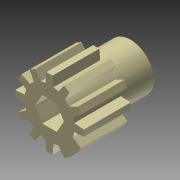
# Autodesk Inventor part: pinion
Saved by Autodesk Inventor 2015 SP1 (Build 190203100, 203)
## iProperties
Created: 2015-01-14
Part Number: pinion
Material: Nylon, molybdenum disulphide
Document SubType Name: Modeling
Designer: Jarod
Density: 1.13 g/cm^3
Appearance: Nylon 6
Author: Jarod
Autodesk Inventor part; units mm, degrees
ref_plane "YZ Plane" through (0, 0, 0) normal (1, 0, 0) x (0, 1, 0)
ref_plane "XZ Plane" through (0, 0, 0) normal (0, 1, 0) x (-1, 0, 0)
ref_plane "XY Plane" through (0, 0, 0) normal (0, 0, 1) x (1, 0, 0)
sketch "Sketch1" plane through (0, 0, 0) normal (0, 0, 1) x (1, 0, 0)
  circle A0 centre (0, 0) radius 11.9062
  dimension "d0" = 23.8125
  constraints: 1 centre point, 1 coincident
  measures "d0" diameter of A0
extrude "Extrusion1" add sketch "Sketch1" along normal blind 41.275
sketch "Sketch2" plane through (0, 0, 41.275) normal (0, 0, 1) x (1, 0, 0)
  circle A0 centre (0, 0) radius 12.7
  dimension "d3" = 25.4
  constraints: 1 centre point, 1 coincident
  measures "d3" diameter of A0
extrude "Extrusion2" add sketch "Sketch2" against normal blind 23.8125
sketch "Sketch3" plane through (0, 0, 41.275) normal (0, 0, 1) x (1, 0, 0)
  line L0 (-3.6662, 6.35) -> (3.6662, 6.35)
  line L1 (3.6662, 6.35) -> (7.3323, 0)
  line L2 (7.3323, 0) -> (3.6662, -6.35)
  line L3 (3.6662, -6.35) -> (-3.6662, -6.35)
  line L4 (-3.6662, -6.35) -> (-7.3323, 0)
  line L5 (-7.3323, 0) -> (-3.6662, 6.35)
  point P0 (0, 0)
  dimension "d6" = 12.7
  dimension "d7" = 12.7
  dimension "d8" = 12.7
  dimension "d9" = 120
  dimension "d10" = 120
  dimension "d11" = 6.35
  dimension "d12" = 6.35
  dimension "d13" = 6.35
  constraints: 12 end point, 3 parallel, 1 horizontal
  measures "d6" distance between parallel lines of L3 L0
  measures "d7" distance between parallel lines of L4 L1
  measures "d8" distance between parallel lines of L2 L5
  measures "d9" angle of L0 L5
  measures "d10" angle of L1 L0
  measures "d11" distance from line of point (0, 0) L0
  measures "d12" distance from line of point (0, 0) L1
  measures "d13" distance from line of point (0, 0) L5
extrude "Extrusion3" cut sketch "Sketch3" against normal blind 50.8
sketch "Sketch4" plane through (0, 0, 41.275) normal (0, 0, 1) x (1, 0, 0)
  line L0 (-7.3323, 0) -> (-3.6662, 6.35) projected
  line L1 (-3.6662, 6.35) -> (3.6662, 6.35) projected
  line L2 (3.6662, 6.35) -> (7.3323, 0) projected
  line L3 (7.3323, 0) -> (3.6662, -6.35) projected
  line L4 (3.6662, -6.35) -> (-3.6662, -6.35) projected
  line L5 (-3.6662, -6.35) -> (-7.3323, 0) projected
  circle A0 centre (0, 0) radius 12.7 projected
  line L6 (0, 12.7) -> (0, 17.4625) construction
  line L7 (0, 12.7) -> (4.7625, 12.7) construction
  line L8 (0, 0) -> (1.9867, 12.5436) construction
  circle A1 centre (0, 0) radius 12.7 construction
  line L9 (0, 0) -> (12.7, 0) construction
  line L10 (0, 0) -> (-1.9867, 12.5436) construction
  line L11 (0, 0) -> (12.7, 0) construction
  line L12 (0, 17.4625) -> (0.7937, 17.4625) construction
  line L13 (0, 17.4625) -> (0.7937, 17.4625) construction
  line L14 (0, 17.4625) -> (-1.5875, 17.4625) construction
  line L15 (0, 17.4625) -> (1.5875, 17.4625) construction
  line L16 (-1.9867, 12.5436) -> (-1.5875, 17.4625)
  line L17 (-1.5875, 17.4625) -> (1.5875, 17.4625)
  line L18 (1.5875, 17.4625) -> (1.9867, 12.5436)
  line L19 (-1.9867, 12.5436) -> (1.9867, 12.5436)
  line L20 (-6.35, 10.9985) -> (-8.7312, 15.123) construction
  line L21 (-6.35, 10.9985) -> (-2.2256, 13.3798) construction
  line L22 (0, 0) -> (-4.5513, 11.8565) construction
  line L23 (0, 0) -> (-7.9924, 9.8698) construction
  line L24 (-8.7312, 15.123) -> (-8.0438, 15.5198) construction
  line L25 (-8.7312, 15.123) -> (-8.0438, 15.5198) construction
  line L26 (-8.7312, 15.123) -> (-10.1061, 14.3292) construction
  line L27 (-8.7312, 15.123) -> (-7.3564, 15.9167) construction
  line L28 (-7.9924, 9.8698) -> (-10.1061, 14.3292)
  line L29 (-10.1061, 14.3292) -> (-7.3564, 15.9167)
  line L30 (-7.3564, 15.9167) -> (-4.5513, 11.8565)
  line L31 (-7.9924, 9.8698) -> (-4.5513, 11.8565)
  line L32 (-10.9985, 6.35) -> (-15.123, 8.7313) construction
  line L33 (-10.9985, 6.35) -> (-8.6173, 10.4744) construction
  line L34 (0, 0) -> (-9.8698, 7.9924) construction
  line L35 (0, 0) -> (-11.8565, 4.5513) construction
  line L36 (-15.123, 8.7313) -> (-14.7261, 9.4187) construction
  line L37 (-15.123, 8.7313) -> (-14.7261, 9.4187) construction
  line L38 (-15.123, 8.7313) -> (-15.9167, 7.3564) construction
  line L39 (-15.123, 8.7313) -> (-14.3292, 10.1061) construction
  line L40 (-11.8565, 4.5513) -> (-15.9167, 7.3564)
  line L41 (-15.9167, 7.3564) -> (-14.3292, 10.1061)
  line L42 (-14.3292, 10.1061) -> (-9.8698, 7.9924)
  line L43 (-11.8565, 4.5513) -> (-9.8698, 7.9924)
  line L44 (-12.7, 0) -> (-17.4625, 0) construction
  line L45 (-12.7, 0) -> (-12.7, 4.7625) construction
  line L46 (0, 0) -> (-12.5436, 1.9867) construction
  line L47 (0, 0) -> (-12.5436, -1.9867) construction
  line L48 (-17.4625, 0) -> (-17.4625, 0.7938) construction
  line L49 (-17.4625, 0) -> (-17.4625, 0.7938) construction
  line L50 (-17.4625, 0) -> (-17.4625, -1.5875) construction
  line L51 (-17.4625, 0) -> (-17.4625, 1.5875) construction
  line L52 (-12.5436, -1.9867) -> (-17.4625, -1.5875)
  line L53 (-17.4625, -1.5875) -> (-17.4625, 1.5875)
  line L54 (-17.4625, 1.5875) -> (-12.5436, 1.9867)
  line L55 (-12.5436, -1.9867) -> (-12.5436, 1.9867)
  line L56 (-10.9985, -6.35) -> (-15.123, -8.7312) construction
  line L57 (-10.9985, -6.35) -> (-13.3798, -2.2256) construction
  line L58 (0, 0) -> (-11.8565, -4.5513) construction
  line L59 (0, 0) -> (-9.8698, -7.9924) construction
  line L60 (-15.123, -8.7312) -> (-15.5198, -8.0438) construction
  line L61 (-15.123, -8.7312) -> (-15.5198, -8.0438) construction
  line L62 (-15.123, -8.7312) -> (-14.3292, -10.1061) construction
  line L63 (-15.123, -8.7312) -> (-15.9167, -7.3564) construction
  line L64 (-9.8698, -7.9924) -> (-14.3292, -10.1061)
  line L65 (-14.3292, -10.1061) -> (-15.9167, -7.3564)
  line L66 (-15.9167, -7.3564) -> (-11.8565, -4.5513)
  line L67 (-9.8698, -7.9924) -> (-11.8565, -4.5513)
  line L68 (-6.35, -10.9985) -> (-8.7313, -15.123) construction
  line L69 (-6.35, -10.9985) -> (-10.4744, -8.6173) construction
  line L70 (0, 0) -> (-7.9924, -9.8698) construction
  line L71 (0, 0) -> (-4.5513, -11.8565) construction
  line L72 (-8.7313, -15.123) -> (-9.4187, -14.7261) construction
  line L73 (-8.7313, -15.123) -> (-9.4187, -14.7261) construction
  line L74 (-8.7313, -15.123) -> (-7.3564, -15.9167) construction
  line L75 (-8.7313, -15.123) -> (-10.1061, -14.3292) construction
  line L76 (-4.5513, -11.8565) -> (-7.3564, -15.9167)
  line L77 (-7.3564, -15.9167) -> (-10.1061, -14.3292)
  line L78 (-10.1061, -14.3292) -> (-7.9924, -9.8698)
  line L79 (-4.5513, -11.8565) -> (-7.9924, -9.8698)
  line L80 (0, -12.7) -> (0, -17.4625) construction
  line L81 (0, -12.7) -> (-4.7625, -12.7) construction
  line L82 (0, 0) -> (-1.9867, -12.5436) construction
  line L83 (0, 0) -> (1.9867, -12.5436) construction
  line L84 (0, -17.4625) -> (-0.7938, -17.4625) construction
  line L85 (0, -17.4625) -> (-0.7938, -17.4625) construction
  line L86 (0, -17.4625) -> (1.5875, -17.4625) construction
  line L87 (0, -17.4625) -> (-1.5875, -17.4625) construction
  line L88 (1.9867, -12.5436) -> (1.5875, -17.4625)
  line L89 (1.5875, -17.4625) -> (-1.5875, -17.4625)
  line L90 (-1.5875, -17.4625) -> (-1.9867, -12.5436)
  line L91 (1.9867, -12.5436) -> (-1.9867, -12.5436)
  line L92 (6.35, -10.9985) -> (8.7312, -15.123) construction
  line L93 (6.35, -10.9985) -> (2.2256, -13.3798) construction
  line L94 (0, 0) -> (4.5513, -11.8565) construction
  line L95 (0, 0) -> (7.9924, -9.8698) construction
  line L96 (8.7312, -15.123) -> (8.0438, -15.5198) construction
  line L97 (8.7312, -15.123) -> (8.0438, -15.5198) construction
  line L98 (8.7312, -15.123) -> (10.1061, -14.3292) construction
  line L99 (8.7312, -15.123) -> (7.3564, -15.9167) construction
  line L100 (7.9924, -9.8698) -> (10.1061, -14.3292)
  line L101 (10.1061, -14.3292) -> (7.3564, -15.9167)
  line L102 (7.3564, -15.9167) -> (4.5513, -11.8565)
  line L103 (7.9924, -9.8698) -> (4.5513, -11.8565)
  line L104 (10.9985, -6.35) -> (15.123, -8.7313) construction
  line L105 (10.9985, -6.35) -> (8.6173, -10.4744) construction
  line L106 (0, 0) -> (9.8698, -7.9924) construction
  line L107 (0, 0) -> (11.8565, -4.5513) construction
  line L108 (15.123, -8.7313) -> (14.7261, -9.4187) construction
  line L109 (15.123, -8.7313) -> (14.7261, -9.4187) construction
  line L110 (15.123, -8.7313) -> (15.9167, -7.3564) construction
  line L111 (15.123, -8.7313) -> (14.3292, -10.1061) construction
  line L112 (11.8565, -4.5513) -> (15.9167, -7.3564)
  line L113 (15.9167, -7.3564) -> (14.3292, -10.1061)
  line L114 (14.3292, -10.1061) -> (9.8698, -7.9924)
  line L115 (11.8565, -4.5513) -> (9.8698, -7.9924)
  line L116 (12.7, 0) -> (17.4625, 0) construction
  line L117 (12.7, 0) -> (12.7, -4.7625) construction
  line L118 (0, 0) -> (12.5436, -1.9867) construction
  line L119 (0, 0) -> (12.5436, 1.9867) construction
  line L120 (17.4625, 0) -> (17.4625, -0.7938) construction
  line L121 (17.4625, 0) -> (17.4625, -0.7938) construction
  line L122 (17.4625, 0) -> (17.4625, 1.5875) construction
  line L123 (17.4625, 0) -> (17.4625, -1.5875) construction
  line L124 (12.5436, 1.9867) -> (17.4625, 1.5875)
  line L125 (17.4625, 1.5875) -> (17.4625, -1.5875)
  line L126 (17.4625, -1.5875) -> (12.5436, -1.9867)
  line L127 (12.5436, 1.9867) -> (12.5436, -1.9867)
  line L128 (10.9985, 6.35) -> (15.123, 8.7313) construction
  line L129 (10.9985, 6.35) -> (13.3798, 2.2256) construction
  line L130 (0, 0) -> (11.8565, 4.5513) construction
  line L131 (0, 0) -> (9.8698, 7.9924) construction
  line L132 (15.123, 8.7313) -> (15.5198, 8.0438) construction
  line L133 (15.123, 8.7313) -> (15.5198, 8.0438) construction
  line L134 (15.123, 8.7313) -> (14.3292, 10.1061) construction
  line L135 (15.123, 8.7313) -> (15.9167, 7.3564) construction
  line L136 (9.8698, 7.9924) -> (14.3292, 10.1061)
  line L137 (14.3292, 10.1061) -> (15.9167, 7.3564)
  line L138 (15.9167, 7.3564) -> (11.8565, 4.5513)
  line L139 (9.8698, 7.9924) -> (11.8565, 4.5513)
  line L140 (6.35, 10.9985) -> (8.7312, 15.123) construction
  line L141 (6.35, 10.9985) -> (10.4744, 8.6173) construction
  line L142 (0, 0) -> (7.9924, 9.8698) construction
  line L143 (0, 0) -> (4.5513, 11.8565) construction
  line L144 (8.7312, 15.123) -> (9.4187, 14.7261) construction
  line L145 (8.7312, 15.123) -> (9.4187, 14.7261) construction
  line L146 (8.7312, 15.123) -> (7.3564, 15.9167) construction
  line L147 (8.7312, 15.123) -> (10.1061, 14.3292) construction
  line L148 (4.5513, 11.8565) -> (7.3564, 15.9167)
  line L149 (7.3564, 15.9167) -> (10.1061, 14.3292)
  line L150 (10.1061, 14.3292) -> (7.9924, 9.8698)
  line L151 (4.5513, 11.8565) -> (7.9924, 9.8698)
  dimension "d16" = 12.7
  dimension "d17" = 0
  dimension "d18" = 4.7625
  dimension "d19" = 90
  dimension "d20" = 81
  dimension "d21" = 99
  dimension "d22" = 0.7937
  dimension "d23" = 0
  dimension "d24" = 1.5875
  dimension "d25" = 180
  dimension "d28" = 360
  constraints: 292 end point, 8 horizontal, 5 equal length, 2 point on circle, 1 vertical, 1 vertical alignment, 277 other
  measures "d16" distance of point (0, 0) L6.start
  measures "d17" horizontal distance of point (0, 0) L6.start
  measures "d18" distance of L6.start L6.end
  measures "d19" angle of L7 L6
  measures "d20" angle of L9 L8
  measures "d21" angle of L11 L10
  measures "d22" distance of L6.end L12.end
  measures "d23" distance between parallel lines of L12 L13
  measures "d24" distance of L6.end L14.end
  measures "d25" angle of L14 L15
extrude "Extrusion4" add sketch "Sketch4" against normal blind 23.8125 contours A0 L127 | A0 L124 L125 L126 | L139 A0 | A0 L136 L137 L138 | L112 L113 L114 A0 | A0 L115 | L151 A0 | A0 L148 L149 L150 | L100 L101 L102 A0 | A0 L103 | L19 A0 | A0 L16 L17 L18 | L88 L89 L90 A0 | A0 L91 | L31 A0 | A0 L28 L29 L30 | L76 L77 L78 A0 | A0 L79 | L43 A0 | A0 L40 L41 L42 | L64 L65 L66 A0 | A0 L67 | L55 A0 | A0 L52 L53 L54
body "Solid1"
